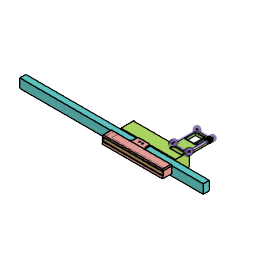
ender revamp (Autodesk Fusion 360 design; units mm, degrees)
Autodesk Fusion 360 part; units mm, degrees
note: some values were not read from the file. Set by a fixed rule: which face or edge a step refers to.
sketch "Sketch1" plane through (0, 0, 0) normal (0, 0, 1) x (1, 0, 0) in component "Component1light bar"
  line L0 (100, -15) -> (-100, -15)
  line L1 (-100, -15) -> (-100, 15)
  line L2 (-100, 15) -> (100, 15)
  line L3 (100, 15) -> (100, -15)
  line L4 (100, -15) -> (-100, 15) construction
  line L5 (-100, -15) -> (100, 15) construction
  line L6 (-33.3333, 15) -> (6.6667, 15)
  line L7 (6.6667, 15) -> (6.6667, 35)
  line L8 (6.6667, 35) -> (-33.3333, 35)
  line L9 (-33.3333, 35) -> (-33.3333, 15)
  circle A0 centre (-18.3333, 25.0583) radius 2.5
  circle A1 centre (-8.3333, 25.0972) radius 2.5
  line L10 (-13.3333, 35) -> (-13.3333, 15) construction
  point P0 (-33.3333, 15)
  point P1 (-33.3333, 25)
  dimension "d1" = 200
  dimension "d2" = 30
  dimension "d3" = 66.6667
  dimension "d4" = 40
  dimension "d5" = 20
  dimension "d6" = 5
  dimension "d7" = 5
  dimension "d8" = 5
  dimension "d9" = 5
  constraint horizontal L0
  constraint perpendicular L0 L1
  constraint parallel L0 L2
  constraint parallel L1 L3
  constraint coincident L4 origin
  constraint coincident L5 origin
  constraint coincident L2 P0
  constraint horizontal L6
  constraint vertical L7
  constraint horizontal L8
  constraint vertical L9
  constraint coincident P0 L6.start
  constraint midpoint L9 P1
  constraint collinear A0.centre A1.centre P1
  constraint midpoint L8 L10.start
  constraint midpoint L6 L10.end
  measures "d1" distance of L1.end L2.end
  measures "d2" distance of L0.end L1.end
  measures "d3" distance of L1.end P0
  measures "d4" distance of P0 L6.end
  measures "d5" distance of P0 L8.end
  measures "d6" diameter of A0
  measures "d7" diameter of A1
  measures "d8" distance of A1.centre L10
  measures "d9" distance of A0.centre L10
extrude "Extrude1" add sketch "Sketch1" against normal blind 20 contours L0 L1 L2 L3 L6 makes body 1 in component "Component1light bar"
extrude "Extrude2" add sketch "Sketch1" against normal blind 5 contours L2 L6 L7 L8 L9 bodies 1 in component "Component1light bar"
fillet "Fillet1" radius 5 2 edges at (-33.3333, 15, -2.5) (6.6667, 15, -2.5) on bodies 1 in component "Component1light bar"
fillet "Fillet2" radius 5 2 edges at (6.6667, 35, -2.5) (-33.3333, 35, -2.5) on bodies 1 in component "Component1light bar"
sketch "Sketch2" plane through (0, -15, 0) normal (0, -1, 0) x (1, 0, 0) in component "Component1light bar"
  line L0 (100, 0) -> (-100, 0)
  line L1 (-100, 0) -> (-100, -20)
  line L2 (-100, -20) -> (100, -20)
  line L3 (100, -20) -> (100, 0)
  line L4 (-90, -2.5) -> (95, -2.5)
  line L5 (95, -2.5) -> (95, -16.5)
  line L6 (95, -16.5) -> (-90, -16.5)
  line L7 (-90, -16.5) -> (-90, -2.5)
  line L8 (100, 0) -> (-100, 0)
  line L9 (-90, -2.5) -> (-76, -2.5)
  line L10 (-76, -2.5) -> (-76, -16.5)
  line L11 (-76, -16.5) -> (-90, -16.5)
  line L12 (-90, -16.5) -> (-90, -2.5)
  line L13 (95, -9.5) -> (-90, -9.5) construction
  dimension "d18" = 5
  dimension "d19" = 10
  dimension "d20" = 3.5
  dimension "d21" = 2.5
  dimension "d22" = 14
  dimension "d25" = 14
  dimension "d26" = 14
  constraint horizontal L4
  constraint vertical L5
  constraint horizontal L6
  constraint vertical L7
  constraint horizontal L9
  constraint vertical L10
  constraint horizontal L11
  constraint vertical L12
  constraint midpoint L5 L13.start
  constraint midpoint L7 L13.end
  measures "d18" distance of L3 L5
  measures "d19" distance of L1 L7
  measures "d20" distance of L2 L6
  measures "d21" distance of L4 L8
  measures "d22" distance of L4.start L6.end
  measures "d25" distance of L4.start L9.end
  measures "d26" distance of L4.start L6.end
extrude "Extrude3" cut sketch "Sketch2" against normal blind 6 contours L4 L6 L7 L9 L10 L11 L12 | L4 L5 L6 L10 bodies 1 in component "Component1light bar"
extrude "Extrude4" cut sketch "Sketch2" against normal blind 69 contours L4 L6 L7 L9 L10 L11 L12 bodies 1 in component "Component1light bar"
fillet "Fillet3" radius 3 1 edges at (-76, -9, -9.5) on bodies 1 in component "Component1light bar"
sketch "Sketch4" plane through (100, 0, 0) normal (1, 0, 0) x (0, 1, 0) in component "Component1light bar"
  line L0 (15, 0) -> (-15, 0)
  line L1 (-15, 0) -> (-15, -20)
  line L2 (-15, -20) -> (15, -20)
  line L3 (15, -20) -> (15, 0)
  line L4 (-15, 0) -> (-18, 0)
  line L5 (-18, 0) -> (-18, -4)
  line L6 (-18, -4) -> (-16.5, -4)
  line L7 (-16.5, -4) -> (-16.5, 0)
  line L8 (-16.5, -2) -> (-15, -2)
  line L9 (-15, -10) -> (-20, -10) construction
  line L10 (-15, -20) -> (-18, -20)
  line L11 (-18, -20) -> (-18, -16)
  line L12 (-18, -16) -> (-16.5, -16)
  line L13 (-16.5, -16) -> (-16.5, -20)
  line L14 (-16.5, -18) -> (-15, -18)
  dimension "d34" = 3
  dimension "d35" = 4
  dimension "d36" = 1.5
  dimension "d37" = 2
  dimension "d38" = 5
  constraint coincident L0.end L1.start
  constraint perpendicular L1 L4
  constraint perpendicular L4 L5
  constraint perpendicular L5 L6
  constraint midpoint L4 L7.end
  constraint coincident L7 L8.start
  constraint coincident L1 L8.end
  constraint perpendicular L1 L8
  constraint midpoint L1 L9.start
  constraint perpendicular L1 L9
  constraint symmetric L0.end L9 L1.end
  constraint symmetric L4.end L9 L10.end
  constraint symmetric L5.end L9 L11.end
  constraint symmetric L6.end L9 L12.end
  constraint symmetric L7.end L9 L13.end
  constraint symmetric L8.start L9 L14.start
  constraint symmetric L8.end L9 L14.end
  measures "d34" distance of L0.end L4.end
  measures "d35" distance of L4.end L5.end
  measures "d36" distance of L5.end L6.end
  measures "d37" distance of L4 L8
  measures "d38" distance of L9.start L9.end
extrude "Extrude5" add sketch "Sketch4" against normal up to surface (200 mm away) contours L1 L4 L7 L8 | L4 L5 L6 L7 | L1 L10 L13 L14 | L10 L11 L12 L13 bodies 1 in component "Component1light bar"
sketch "Sketch5" plane through (-100, 0, 0) normal (-1, 0, 0) x (0, -1, 0) in component "Component1light bar"
  line L0 (18, 0) -> (-15, 0)
  line L1 (-15, 0) -> (-15, -20)
  line L2 (-15, -20) -> (18, -20)
  line L3 (18, -20) -> (18, -16)
  line L4 (18, -16) -> (16.5, -16)
  line L5 (16.5, -16) -> (16.5, -18)
  line L6 (16.5, -18) -> (15, -18)
  line L7 (15, -18) -> (15, -2)
  line L8 (15, -2) -> (16.5, -2)
  line L9 (16.5, -2) -> (16.5, -4)
  line L10 (16.5, -4) -> (18, -4)
  line L11 (18, -4) -> (18, 0)
  line L12 (18, 0) -> (11.8018, 0)
  line L13 (11.8018, 0) -> (11.8018, -20)
  line L14 (11.8018, -20) -> (18, -20)
  line L15 (18, -20) -> (18, 0)
  constraint horizontal L12
  constraint vertical L13
  constraint horizontal L14
  constraint vertical L15
  constraint coincident L2 L13.end
  constraint coincident L0.start L11.end
extrude "Extrude6" add sketch "Sketch5" against normal blind 5 contours L0 L2 L3 L4 L5 L6 L7 L8 L9 L10 L11 L12 L13 L14 L15 | L4 L5 L6 L7 L8 L9 L10 L15 bodies 1 in component "Component1light bar"
sketch "Sketch1 (2)" plane through (100, 0, 0) normal (1, 0, 0) x (0, 1, 0) in component "diffuser"
  line L0 (15, 0) -> (-18, 0)
  line L1 (-18, 0) -> (-18, -4)
  line L2 (-18, -4) -> (-16.5, -4)
  line L3 (-16.5, -4) -> (-16.5, -2)
  line L4 (-16.5, -2) -> (-15, -2)
  line L5 (-15, -2) -> (-15, -18)
  line L6 (-15, -18) -> (-16.5, -18)
  line L7 (-16.5, -18) -> (-16.5, -16)
  line L8 (-16.5, -16) -> (-18, -16)
  line L9 (-18, -16) -> (-18, -20)
  line L10 (-18, -20) -> (15, -20)
  line L11 (15, -20) -> (15, 0)
  line L12 (-18, -4.4) -> (-16.1, -4.4)
  line L13 (-16.1, -4.4) -> (-16.1, -2.4)
  line L14 (-16.1, -2.4) -> (-15.4, -2.4)
  line L15 (-15.4, -2.4) -> (-15.4, -17.6)
  line L16 (-15.4, -17.6) -> (-16.1, -17.6)
  line L17 (-16.1, -17.6) -> (-16.1, -15.6)
  line L18 (-16.1, -15.6) -> (-18, -15.6)
  line L19 (-18, -4.4) -> (-18, -15.6)
  dimension "d43" = 0.4
  constraint perpendicular L12 L19
extrude "Extrude1'" add sketch "Sketch1 (2)" against normal up to surface (195 mm away) separate body contours L12 L13 L14 L15 L16 L17 L18 L19 makes body 2 in component "diffuser"
split "Split1" by plane through (6.6667, 15, 0) normal (0, 1, 0) bodies 1 makes body 3 at (-11.8521, 32.5115, 0) in component "Component1light bar"
sketch "Sketch1 (1)" plane through (0, 15, 0) normal (0, 1, 0) x (-1, 0, 0) in component "Component1light bar"
  line L0 (76, -16.5) -> (76, -2.5)
  line L1 (76, -2.5) -> (90, -2.5)
  line L2 (90, -2.5) -> (90, -16.5)
  line L3 (90, -16.5) -> (76, -16.5)
  line L4 (100, 0) -> (-100, 0)
  line L5 (-100, 0) -> (-100, -20)
  line L6 (-100, -20) -> (100, -20)
  line L7 (100, -20) -> (100, 0)
  line L8 (38.3333, 0) -> (-11.6667, 0)
  line L9 (38.3333, -5) -> (38.3333, 0)
  line L10 (38.3333, -5) -> (-11.6667, -5)
  line L11 (-11.6667, 0) -> (-11.6667, -5)
extrude "Extrude1''" cut sketch "Sketch1 (1)" against normal blind 3 contours L4 L8 L9 L10 L11 bodies 1 in component "Component1light bar"
extrude "Extrude2'" add 1 faces at (-21.6667, 15, -1.6667) along direction (0, -1, 0) blind 3 on bodies 3 bodies 3 in component "Component1light bar"
fillet "Fillet1'" radius 3 5 edges at (-69.1667, 15, 0) (-100, -1.5, 0) (0, -18, 0) (55.8333, 15, 0) (100, -1.5, 0) on bodies 1 in component "Component1light bar"
fillet "Fillet2'" radius 3 6 edges at (-99.1213, -17.1213, -0.8787) (-100, -18, -11.5) (99.1213, 14.1213, -0.8787) (100, 15, -11.5) (-99.1213, 14.1213, -0.8787) (-100, 15, -11.5) on bodies 1 in component "Component1light bar"
sketch "Sketch2 (1)" plane through (0, 0, -20) normal (0, 0, -1) x (1, 0, 0) in component "Component1light bar"
  line L0 (-92, 12) -> (92, 12)
  line L1 (92, 12) -> (92, -9)
  line L2 (92, -9) -> (-92, -9)
  line L3 (-92, -9) -> (-92, 12)
  line L4 (100, 15) -> (-100, 15)
  line L5 (-76, 6) -> (-76, -15)
  line L6 (-90, 15) -> (-90, -15)
  line L7 (-92, 12) -> (-76, 12)
  line L8 (-76, 12) -> (-76, -9)
  line L9 (-76, -9) -> (-92, -9)
  line L10 (-92, -9) -> (-92, 12)
  arc A0 (-100, -12) -> (-97, -15) centre (-97, -12) ccw
  line L11 (-97, -15) -> (97, -15)
  arc A1 (97, -15) -> (100, -12) centre (97, -12) ccw
  line L12 (100, -12) -> (100, 18)
  line L13 (100, 18) -> (-97, 18)
  arc A2 (-97, 18) -> (-100, 15) centre (-97, 15) ccw
  line L14 (-100, 15) -> (-100, -12)
  dimension "d59" = 3
  constraint horizontal L0
  constraint vertical L1
  constraint horizontal L2
  constraint vertical L3
  constraint horizontal L7
  constraint vertical L8
  constraint horizontal L9
  constraint vertical L10
  constraint coincident L5 L8.end
  constraint coincident L2 L8.end
  measures "d59" distance of L0 L4
extrude "Extrude4'" add sketch "Sketch2 (1)" along normal blind 5 contours L0 L1 L2 L4 L5 L6 L7 L11 A1 L12 | L0 L2 L3 L4 L6 L7 L9 L10 A0 L11 L14 | L4 L12 L13 A2 | L2 L5 L6 L9 L11 bodies 1 in component "Component1light bar"
extrude "Extrude5'" cut sketch "Sketch2 (1)" against normal up to surface (3.5 mm away) contours L0 L2 L5 L6 L7 L8 L9 | L0 L2 L3 L6 L7 L9 L10 bodies 1 in component "Component1light bar"
fillet "Fillet4" radius 3 1 edges at (-90, -15, -9.5) on bodies 1 in component "Component1light bar"
sketch "Sketch1 (3)" plane through (-100, 0, 0) normal (-1, 0, 0) x (0, -1, 0) in component "top bar"
  line L0 (-12, -3) -> (-12, -25)
  line L1 (-12, -25) -> (15, -25)
  line L2 (15, -25) -> (15, -3)
  line L3 (15, -3) -> (-12, -3)
  line L4 (-12, -25) -> (-12, -3)
  line L5 (-15, -3) -> (-12, -3)
  line L6 (-15, -3) -> (-15, -25)
  line L7 (-15, -25) -> (-12, -25)
  line L8 (-15, -25) -> (-35, -25)
  line L9 (-35, -25) -> (-35, 5)
  line L10 (-35, 5) -> (-15, 5)
  line L11 (-15, 5) -> (-15, -25)
  dimension "d68" = 20
  dimension "d69" = 30
  constraint horizontal L8
  constraint vertical L9
  constraint horizontal L10
  constraint vertical L11
  constraint coincident L6.end L7.start
  measures "d68" distance of L6.end L8.end
  measures "d69" distance of L6.end L10.end
extrude "Extrude1'''" add sketch "Sketch1 (3)" along normal mid plane 600 separate body contours L6 L8 L9 L10 L11 makes body 4 in component "top bar"
move_body "Move1" bodies 4 to x (1, 0, 0) y (0, 1, 0) z (0, 0, 1) at (0, 0, -10) in component "top bar"
sketch "Sketch1 (4)" plane through (0, 35, 0) normal (0, 1, 0) x (-1, 0, 0) in component "pi_holder"
  line L0 (-200, -35) -> (400, -35)
  line L1 (400, -35) -> (400, -5)
  line L2 (400, -5) -> (-200, -5)
  line L3 (-200, -5) -> (-200, -35)
  line L4 (-85.6295, -5) -> (89.3705, -5)
  line L5 (89.3705, -5) -> (89.3705, -45)
  line L6 (89.3705, -45) -> (-85.6295, -45)
  line L7 (-85.6295, -45) -> (-85.6295, -5)
  dimension "d72" = 175
  dimension "d73" = 40
  constraint horizontal L4
  constraint vertical L5
  constraint horizontal L6
  constraint vertical L7
  constraint coincident L2 L4.start
  measures "d72" distance of L4.start L4.end
  measures "d73" distance of L4.start L6.end
extrude "Extrude1''''" add sketch "Sketch1 (4)" along normal blind 40 separate body contours L0 L2 L4 L5 L7 | L0 L5 L6 L7 makes body 5 in component "pi_holder"
shell "Shell1" thickness 3 outward yes removed faces 2 at (-89.3705, 61.6667, -38.3333) at (-89.3705, 61.6667, -15) on bodies 5 in component "pi_holder"
move_body "Move1'" bodies 5 to x (1, 0, 0) y (0, 1, 0) z (0, 0, 1) at (0, 3, 0) in component "pi_holder"
fillet "Fillet1''" radius 5 2 edges at (-0.3705, 81, -2) (-0.3705, 81, -48) on bodies 5 in component "pi_holder"
fillet "Fillet2''" radius 5 2 edges at (-1.8705, 78, -45) (-1.8705, 78, -5) on bodies 5 in component "pi_holder"
sketch "Sketch3" plane through (88.6295, 0, 0) normal (1, 0, 0) x (0, 1, 0) in component "pi_holder"
  arc A0 (76, -48) -> (81, -43) centre (76, -43) ccw
  line L0 (81, -43) -> (81, -7)
  arc A1 (81, -7) -> (76, -2) centre (76, -7) ccw
  line L1 (76, -2) -> (35, -2)
  line L2 (35, -2) -> (35, -48)
  line L3 (35, -48) -> (76, -48)
  line L4 (76, -2) -> (156, -2)
  line L5 (156, -2) -> (156, -12)
  line L6 (156, -12) -> (76, -12)
  line L7 (76, -12) -> (76, -2)
  dimension "d83" = 80
  dimension "d84" = 10
  constraint horizontal L4
  constraint vertical L5
  constraint horizontal L6
  constraint vertical L7
  constraint coincident A1.end L1.start
  measures "d83" distance of A1.end L4.end
  measures "d84" distance of A1.end L6.end
extrude "Extrude2''" add sketch "Sketch3" against normal blind 50 separate body contours L0 A1 L4 L5 L6 makes body 6 in component "pi_holder"
sketch "Sketch5 (2)" plane through (0, 0, -2) normal (0, 0, 1) x (-1, 0, 0) in component "pi_holder"
  line L0 (-88.6295, -76) -> (89.3705, -76)
  line L1 (89.3705, -76) -> (89.3705, -35)
  line L2 (89.3705, -35) -> (-88.6295, -35)
  line L3 (-88.6295, -35) -> (-88.6295, -76)
  line L4 (89.3705, -76) -> (89.3705, -81)
  line L5 (89.3705, -81) -> (-88.6295, -81)
  line L6 (-88.6295, -81) -> (-88.6295, -76)
  line L7 (-88.6295, -35) -> (-88.6295, -76)
  line L8 (89.3705, -35) -> (89.3705, -76)
  line L9 (89.3705, -35) -> (-88.6295, -35)
  line L10 (-85.6295, -73) -> (-45.6295, -73)
  line L11 (-45.6295, -73) -> (-45.6295, -58)
  line L12 (-45.6295, -58) -> (-85.6295, -58)
  line L13 (-85.6295, -58) -> (-85.6295, -73)
  dimension "d87" = 40
  dimension "d88" = 15
  dimension "d89" = 3
  dimension "d90" = 3
  constraint horizontal L10
  constraint vertical L11
  constraint horizontal L12
  constraint vertical L13
  measures "d87" distance of L10.start L10.end
  measures "d88" distance of L10.start L12.end
  measures "d89" distance of L7 L13
  measures "d90" distance of L0 L10
extrude "Extrude3'" cut sketch "Sketch5 (2)" against normal blind 5 contours L10 L11 L12 L13 bodies 5 in component "pi_holder"
fillet "Fillet3'" radius 3 4 edges at (45.6295, 58, -3.5) (45.6295, 73, -3.5) (85.6295, 58, -3.5) (85.6295, 73, -3.5) on bodies 5 in component "pi_holder"
sketch "Sketch6" plane through (0, 0, -2) normal (0, 0, 1) x (-1, 0, 0) in component "pi_holder"
  line L0 (-88.6295, -76) -> (-88.6295, -156)
  line L1 (-88.6295, -156) -> (-38.6295, -156)
  line L2 (-38.6295, -156) -> (-38.6295, -76)
  line L3 (-38.6295, -76) -> (-88.6295, -76)
  line L4 (-88.6295, -76) -> (-38.6295, -76)
  line L5 (-88.6295, -81) -> (-88.6295, -76)
  line L6 (-38.6295, -81) -> (-38.6295, -76)
  line L7 (-88.6295, -156) -> (-88.6295, -81)
  line L8 (-38.6295, -156) -> (-38.6295, -81)
  line L9 (-88.6295, -156) -> (-38.6295, -156)
  line L10 (-83.6295, -146) -> (-43.6295, -146)
  line L11 (-43.6295, -146) -> (-43.6295, -111)
  line L12 (-43.6295, -111) -> (-83.6295, -111)
  line L13 (-83.6295, -111) -> (-83.6295, -146)
  line L14 (-73.6295, -111) -> (-88.6295, -111)
  line L15 (-88.6295, -111) -> (-88.6295, -146)
  line L16 (-88.6295, -146) -> (-73.6295, -146)
  line L17 (-73.6295, -146) -> (-73.6295, -111)
  line L18 (-85.6295, -143) -> (-76.6295, -143)
  line L19 (-76.6295, -143) -> (-76.6295, -114)
  line L20 (-76.6295, -114) -> (-85.6295, -114)
  line L21 (-85.6295, -114) -> (-85.6295, -143)
  dimension "d95" = 40
  dimension "d96" = 35
  dimension "d97" = 5
  dimension "d98" = 5
  dimension "d99" = 10
  dimension "d104" = 35
  dimension "d105" = 15
  dimension "d106" = -3
  constraint horizontal L10
  constraint vertical L11
  constraint horizontal L12
  constraint vertical L13
  constraint horizontal L14
  constraint vertical L15
  constraint horizontal L16
  constraint vertical L17
  constraint coincident L0 L15.end
  constraint coincident L12 L14.start
  measures "d95" distance of L10.start L10.end
  measures "d96" distance of L10.start L12.end
  measures "d97" distance of L7 L13
  measures "d98" distance of L8 L11
  measures "d99" distance of L9 L10
  measures "d104" distance of L14.start L16.end
  measures "d105" distance of L14.start L14.end
extrude "Extrude4''" cut sketch "Sketch6" against normal blind 145 contours L10 L12 L13 L14 L16 L17 L18 L19 L20 | L10 L11 L12 L17 | L13 L18 L19 L20 bodies 6 in component "pi_holder"
extrude "Extrude5''" cut sketch "Sketch6" against normal blind 35 contours L13 L18 L19 L20 | L13 L18 L20 L21 bodies 6 in component "pi_holder"
extrude "Extrude6'" add sketch "Sketch6" against normal up to surface (10 mm away) contours L10 L12 L13 L14 L16 L17 L18 L19 L20 bodies 6 in component "pi_holder"
fillet "Fillet4'" radius 5 2 edges at (88.6295, 156, -7) (38.6295, 156, -7) on bodies 6 in component "pi_holder"
fillet "Fillet5" radius 3 5 edges at (88.6295, 113.5, -2) (87.165, 154.5355, -2) (63.6295, 156, -2) (40.0939, 154.5355, -2) (38.6295, 113.5, -2) on bodies 6 in component "pi_holder"
fillet "Fillet6" radius 1 4 edges at (43.6295, 128.5, -2) (58.6295, 146, -2) (73.6295, 128.5, -2) (58.6295, 111, -2) on bodies 6 in component "pi_holder"
component "Component1light bar" placed x (1, 0, 0) y (0, 1, 0) z (0, 0, 1) at (0, 0, 0)
component "top bar" placed x (1, 0, 0) y (0, 1, 0) z (0, 0, 1) at (0, 0, 0)
component "pi_holder" placed x (1, 0, 0) y (0, 1, 0) z (0, 0, 1) at (0, 0, 0)
component "diffuser" placed x (1, 0, 0) y (0, 1, 0) z (0, 0, 1) at (0, 0, 0) in component "Component1light bar"
equation "d3 = ( 200 / 3 ) * 1 mm"
named bodies: "lip"
